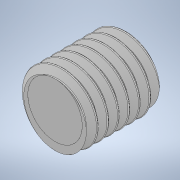
# Autodesk Inventor part: thread-m
Saved by Autodesk Inventor 2022 (Build 260153000, 153)
## iProperties
Created: 2021-10-07
Part Number: thread-m
Material: Generic
Document SubType Name: Modeling
Designer: tecware
Density: 1 g/cm^3
Appearance: Default
Author: tecware
## iProperties of the stored document thread-m_3DPrint.ipt
Created: 2021-10-07
Part Number: thread-m_3DPrint
Material: Generic
Document SubType Name: Modeling
Designer: tecware
Density: 1 g/cm^3
Appearance: Default
Author: tecware
Autodesk Inventor part; units mm, degrees
ref_plane "YZ Plane" through (0, 0, 0) normal (1, 0, 0) x (0, 1, 0)
ref_plane "XZ Plane" through (0, 0, 0) normal (0, 1, 0) x (-1, 0, 0)
ref_plane "XY Plane" through (0, 0, 0) normal (0, 0, 1) x (1, 0, 0)
sketch "Sketch1" plane through (0, 0, 0) normal (0, 0, 1) x (1, 0, 0)
  circle A0 centre (0, 0) radius 5
  dimension "d0" = 10
  constraints: 1 centre point, 1 coincident
  measures "d0" diameter of A0
extrude "Extrusion1" add sketch "Sketch1" along normal blind 10
thread "Thread1" size "M10x1.5" class "6g" standard "ANSI Metric M Profile" full length
sketch "Sketch3" plane through (0, 0, 10) normal (-1, 0, 0) x (0, 1, 0)
  line L0 (5, 0) -> (5, 10)
  line L1 (5, 10) -> (3.8878, 10)
  line L2 (3.8878, 10) -> (3.8878, 0)
  line L3 (3.8878, 0) -> (5, 0)
  line L4 (0, -3.9629) -> (0, 12.3271) projected
  constraints: 8 end point
revolve "Revolution1" cut sketch "Sketch3" angle 360 about axis through (0, 0, 10) along (0, 0, -1)
sketch "Sketch4" plane through (0, 0, 10) normal (-1, 0, 0) x (0, 1, 0)
  line L0 (5, 0) -> (5, 10)
  line L1 (5, 10) -> (3.8878, 10)
  line L2 (3.8878, 10) -> (3.8878, 0)
  line L3 (3.8878, 0) -> (5, 0)
  line L4 (0, -3.9629) -> (0, 12.3271) projected
  constraints: 8 end point
revolve "Revolution2" add sketch "Sketch4" angle 360 about axis through (0, 0, 10) along (0, 0, -1) separate body
sketch "Sketch2" plane through (0, 0, 10) normal (1, 0, 0) x (0, 0, -1)
  line L0 (-0.8751, -3.9638) -> (-0.7501, -3.9638) construction
  line L1 (0.1249, -4.9243) -> (-0.0001, -5.1644) construction
  line L2 (-1.5001, -5.1644) -> (-1.6251, -4.9243) construction
  line L3 (-0.6251, -3.9638) -> (-0.7501, -3.7237) construction
  line L4 (-0.7501, -3.7237) -> (-0.8751, -3.9638) construction
  line L5 (-1.5001, -5.1644) -> (-1.3751, -4.9243) construction
  line L6 (-0.6251, -3.9638) -> (-0.1251, -4.9243)
  line L7 (-1.6251, -4.9243) -> (-1.3751, -4.9243) construction
  arc A0 (-1.6251, -4.9243) -> (-1.5001, -5.0002) centre (-1.5001, -4.8592) ccw construction
  line L8 (0.1249, -4.9243) -> (-0.1251, -4.9243) construction
  line L9 (-1.5001, -5.1644) -> (-1.5001, -4.9243) construction
  line L10 (-0.0001, -5.1644) -> (-0.0001, -4.9243) construction
  line L11 (-0.7501, -3.7237) -> (-0.7501, -3.888) construction
  line L12 (-1.5001, -5.0002) -> (-0.0001, -5.0002)
  arc A1 (-1.5001, -5.0002) -> (-1.3751, -4.9243) centre (-1.5001, -4.8592) ccw
  line L13 (-0.1251, -4.9243) -> (-0.0001, -5.1644) construction
  line L14 (-1.3751, -4.9243) -> (-0.8751, -3.9638)
  line L15 (-0.0001, -0.0002) -> (-0.0001, 0.0177)
  line L16 (-0.0001, 0.0177) -> (-0.0001, -0.0002)
  line L17 (-0.0001, -0.0002) -> (0.0334, -0.0002)
  arc A2 (-0.1251, -4.9243) -> (-0.0001, -5.0002) centre (-0.0001, -4.8592) ccw
  arc A3 (-0.0001, -5.0002) -> (0.1249, -4.9243) centre (-0.0001, -4.8592) ccw construction
  arc A4 (-0.7501, -3.888) -> (-0.8751, -3.9638) centre (-0.7501, -4.0289) ccw
  arc A5 (-0.6251, -3.9638) -> (-0.7501, -3.888) centre (-0.7501, -4.0289) ccw
  line L18 (-0.7501, -3.888) -> (-0.7501, -3.9638) construction
  line L19 (-0.7501, -3.9638) -> (-0.6251, -3.9638) construction
  dimension "d5" = 55
  dimension "d6" = 0.2401
  dimension "d7" = 0.2401
  dimension "Sketch2_ThreadOffset" = 0
  dimension "Sketch2_MajorRadius" = 5
  dimension "d10" = 1.5
  dimension "Sketch2_MinorRadius" = 3.8878
  constraints: 40 end point, 12 point on circle, 10 parallel, 8 tangent, 6 centre point, 6 collinear, 2 midpoint, 2 point on line, 1 horizontal, 1 perpendicular, 3 other
  measures "d5" angle of L6 L14
  measures "d6" distance of L3.end L0.end
  measures "d7" distance of L1.end L10.end
  measures "Sketch2_ThreadOffset" distance between parallel lines of L15 L10
  measures "Sketch2_MajorRadius" distance from line of L12 L15.start
  measures "d10" distance from line of L1.end L9
  measures "Sketch2_MinorRadius" distance edge to line of A5 L17
coil "Coil1" sketch "Sketch2" operation cut axis through (0, 0, 10) along (0, 0, -1) pitch 1.5015 turns 8.658009 hand right bodies 2
equation "\"d5\" = d12"
equation "\"d6\" = 0.160083 * Sketch2_Pitch"
equation "\"d7\" = 0.160083 * Sketch2_Pitch"
equation "\"d10\" = Sketch2_Pitch"
equation "\"d12\" = 55deg"
equation "\"Sketch2_Pitch\" = 1.5"
body "Solid1"
body "Solid2"
